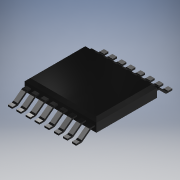
# Autodesk Inventor part: 16_pin_IC
Saved by Autodesk Inventor 2017 SP1 (Build 210196100, 196)
## iProperties
Created: 2016-08-29
Part Number: 16_pin_IC
Material: PBT Plastic
Document SubType Name: Modeling
Designer: jwrjc
Density: 1.31 g/cm^3
Appearance: Smooth - White
Author: jwrjc
Autodesk Inventor part; units mm, degrees
ref_plane "YZ Plane" through (0, 0, 0) normal (1, 0, 0) x (0, 1, 0)
ref_plane "XZ Plane" through (0, 0, 0) normal (0, 1, 0) x (-1, 0, 0)
ref_plane "XY Plane" through (0, 0, 0) normal (0, 0, 1) x (1, 0, 0)
sketch "Sketch1" plane through (0, 0, 0) normal (0, 0, 1) x (1, 0, 0)
  line L0 (-6.1646, -19.4392) -> (-11.1748, -19.4392)
  line L1 (-11.1748, -19.4392) -> (-11.1748, -23.673)
  line L2 (-11.1748, -23.673) -> (-6.1646, -23.673)
  line L3 (-6.1646, -23.673) -> (-6.1646, -19.4392)
  line L4 (-6.5748, -19.4392) -> (-6.2818, -19.4392)
  line L5 (-6.2818, -19.4392) -> (-6.2818, -18.2673)
  line L6 (-6.2818, -18.2673) -> (-6.5748, -18.2673)
  line L7 (-6.5748, -18.2673) -> (-6.5748, -19.4392)
  line L8 (-7.2047, -19.4392) -> (-6.8971, -19.4392)
  line L9 (-6.8971, -19.4392) -> (-6.8971, -18.2673)
  line L10 (-6.8971, -18.2673) -> (-7.2047, -18.2673)
  line L11 (-7.2047, -18.2673) -> (-7.2047, -19.4392)
  line L12 (-7.8347, -19.4392) -> (-7.5124, -19.4392)
  line L13 (-7.5124, -19.4392) -> (-7.5124, -18.2673)
  line L14 (-7.5124, -18.2673) -> (-7.8347, -18.2673)
  line L15 (-7.8347, -18.2673) -> (-7.8347, -19.4392)
  line L16 (-8.4939, -19.4392) -> (-8.1716, -19.4392)
  line L17 (-8.1716, -19.4392) -> (-8.1716, -18.2673)
  line L18 (-8.1716, -18.2673) -> (-8.4939, -18.2673)
  line L19 (-8.4939, -18.2673) -> (-8.4939, -19.4392)
  line L20 (-9.1824, -19.4392) -> (-8.8455, -19.4392)
  line L21 (-8.8455, -19.4392) -> (-8.8455, -18.2673)
  line L22 (-8.8455, -18.2673) -> (-9.1824, -18.2673)
  line L23 (-9.1824, -18.2673) -> (-9.1824, -19.4392)
  line L24 (-9.8124, -19.4392) -> (-9.4754, -19.4392)
  line L25 (-9.4754, -19.4392) -> (-9.4754, -18.2673)
  line L26 (-9.4754, -18.2673) -> (-9.8124, -18.2673)
  line L27 (-9.8124, -18.2673) -> (-9.8124, -19.4392)
  line L28 (-10.4569, -19.4392) -> (-10.1347, -19.4392)
  line L29 (-10.1347, -19.4392) -> (-10.1347, -18.2673)
  line L30 (-10.1347, -18.2673) -> (-10.4569, -18.2673)
  line L31 (-10.4569, -18.2673) -> (-10.4569, -19.4392)
  line L32 (-11.0429, -19.4392) -> (-10.7353, -19.4392)
  line L33 (-10.7353, -19.4392) -> (-10.7353, -18.2673)
  line L34 (-10.7353, -18.2673) -> (-11.0429, -18.2673)
  line L35 (-11.0429, -18.2673) -> (-11.0429, -19.4392)
  line L36 (-11.0429, -23.673) -> (-10.7353, -23.673)
  line L37 (-10.7353, -23.673) -> (-10.7353, -24.9622)
  line L38 (-10.7353, -24.9622) -> (-11.0429, -24.9622)
  line L39 (-11.0429, -24.9622) -> (-11.0429, -23.673)
  line L40 (-10.4569, -23.673) -> (-10.1347, -23.673)
  line L41 (-10.1347, -23.673) -> (-10.1347, -24.9622)
  line L42 (-10.1347, -24.9622) -> (-10.4569, -24.9622)
  line L43 (-10.4569, -24.9622) -> (-10.4569, -23.673)
  line L44 (-9.8124, -23.673) -> (-9.4754, -23.673)
  line L45 (-9.4754, -23.673) -> (-9.4754, -24.9622)
  line L46 (-9.4754, -24.9622) -> (-9.8124, -24.9622)
  line L47 (-9.8124, -24.9622) -> (-9.8124, -23.673)
  line L48 (-9.1824, -23.673) -> (-8.8455, -23.673)
  line L49 (-8.8455, -23.673) -> (-8.8455, -24.9622)
  line L50 (-8.8455, -24.9622) -> (-9.1824, -24.9622)
  line L51 (-9.1824, -24.9622) -> (-9.1824, -23.673)
  line L52 (-8.4939, -23.673) -> (-8.1716, -23.673)
  line L53 (-8.1716, -23.673) -> (-8.1716, -24.9622)
  line L54 (-8.1716, -24.9622) -> (-8.4939, -24.9622)
  line L55 (-8.4939, -24.9622) -> (-8.4939, -23.673)
  line L56 (-7.8347, -23.673) -> (-7.5124, -23.673)
  line L57 (-7.5124, -23.673) -> (-7.5124, -24.9622)
  line L58 (-7.5124, -24.9622) -> (-7.8347, -24.9622)
  line L59 (-7.8347, -24.9622) -> (-7.8347, -23.673)
  line L60 (-7.2047, -23.673) -> (-6.8971, -23.673)
  line L61 (-6.8971, -23.673) -> (-6.8971, -24.9622)
  line L62 (-6.8971, -24.9622) -> (-7.2047, -24.9622)
  line L63 (-7.2047, -24.9622) -> (-7.2047, -23.673)
  line L64 (-6.5748, -23.673) -> (-6.2818, -23.673)
  line L65 (-6.2818, -23.673) -> (-6.2818, -24.9622)
  line L66 (-6.2818, -24.9622) -> (-6.5748, -24.9622)
  line L67 (-6.5748, -24.9622) -> (-6.5748, -23.673)
  point P0 (0, 0)
  constraints: 132 end point, 33 parallel, 30 point on line, 16 horizontal, 16 perpendicular, 1 vertical, 22 other
extrude "Extrusion1" add sketch "Sketch1" along normal blind 1 contours L3 L2 L1 L0
extrude "Extrusion2" add sketch "Sketch1" along normal blind 0.6 contours L0 L7 L6 L5 | L65 L66 L67 L2 | L0 L11 L10 L9 | L61 L62 L63 L2 | L0 L15 L14 L13 | L57 L58 L59 L2 | L0 L19 L18 L17 | L53 L54 L55 L2 | L0 L23 L22 L21 | L49 L50 L51 L2 | L0 L27 L26 L25 | L45 L46 L47 L2 | L0 L31 L30 L29 | L41 L42 L43 L2 | L0 L35 L34 L33 | L37 L38 L39 L2
sketch "Sketch2" plane through (-11.0429, -19.4392, 0) normal (-1, 0, 0) x (0, 0, 1)
  line L0 (0, 0) -> (0, 1.172) projected
  line L1 (0.6, 1.172) -> (0.1113, 1.172)
  line L2 (0, 0) -> (0.599, 0)
  line L3 (0.6, 0.3044) -> (0.6, 1.172)
  line L4 (0.6, -4.2338) -> (0.6, -5.5229) projected
  line L5 (0, -4.2338) -> (0, -5.5229) projected
  line L6 (0.5, -4.2338) -> (0, -4.2338)
  line L7 (0, -4.2338) -> (0, -5.1366)
  line L8 (0.1113, -5.5229) -> (0.6, -5.5229)
  line L9 (0.6, -5.5229) -> (0.6, -4.5423)
  line L10 (0, 1.172) -> (0.6, 1.172) projected
  line L11 (0.1113, 1.172) -> (0.1113, 0.7931)
  line L12 (0.1113, 0.7931) -> (0.6, 0.3044)
  line L13 (0.6, 0) -> (0.6, 1.172) projected
  line L14 (0.6, 0) -> (0.5, 0)
  line L15 (0, 0) -> (1, 0) projected
  line L16 (0.5, 0) -> (0.5, 0.2353)
  line L17 (0.5, 0.2353) -> (0, 0.7353)
  line L18 (0, -5.5229) -> (0.6, -5.5229) projected
  line L19 (0.1113, -5.5229) -> (0.1113, -5.1962)
  line L20 (0.1113, -5.1962) -> (0.6, -4.5423)
  line L21 (0.6, -4.2338) -> (0.6, -4.2828)
  line L22 (0, -4.2338) -> (1, -4.2338) projected
  line L23 (0.5, -4.2338) -> (0.5, -4.4676)
  line L24 (0.5, -4.4676) -> (0, -5.1366)
  line L25 (0, 1.1726) -> (0, 1.172)
  line L26 (0, 0.7353) -> (0, 0)
  line L27 (0, 0.7353) -> (0.5, 0.2353)
  line L28 (0.5, 0.2353) -> (0.5, 0)
  line L29 (0.5, 0) -> (0, 0)
  line L30 (0, 0) -> (0, 0.7353)
  point P0 (0, 19.4392)
  constraints: 47 end point, 10 point on line, 7 parallel, 4 perpendicular, 3 collinear, 2 horizontal, 2 midpoint, 2 vertical
extrude "Extrusion3" cut sketch "Sketch2" against normal blind 4.9 contours L0 L17 L16 L2 | L1 L3 L12 L11 | L23 L24 L5 L6 | L4 L8 L19 L20
fillet "Fillet1" radius 0.2 64 edges at (-6.4283, -18.6461, 0.1113) (-7.0509, -18.6461, 0.1113) (-7.6735, -18.6461, 0.1113) (-8.3327, -18.6461, 0.1113) (-9.014, -18.6461, 0.1113) (-9.6439, -18.6461, 0.1113) (-10.2958, -18.6461, 0.1113) (-10.8891, -18.6461, 0.1113) (-10.8891, -19.1348, 0.6) (-10.2958, -19.1348, 0.6) (-9.6439, -19.1348, 0.6) (-9.014, -19.1348, 0.6) (-8.3327, -19.1348, 0.6) (-7.6735, -19.1348, 0.6) (-7.0509, -19.1348, 0.6) (-6.4283, -19.1348, 0.6) (-6.4283, -23.9816, 0.6) (-7.0509, -23.9816, 0.6) (-7.6735, -23.9816, 0.6) (-8.3327, -23.9816, 0.6) (-9.014, -23.9816, 0.6) (-9.6439, -23.9816, 0.6) (-10.2958, -23.9816, 0.6) (-10.8891, -23.9816, 0.6) (-10.8891, -23.9068, 0.5) (-10.2958, -23.9068, 0.5) (-9.6439, -23.9068, 0.5) (-9.014, -23.9068, 0.5) (-8.3327, -23.9068, 0.5) (-7.6735, -23.9068, 0.5) (-7.0509, -23.9068, 0.5) (-6.4283, -23.9068, 0.5) (-6.4283, -24.6354, 0.1113) (-6.4283, -24.5758, 0) (-7.0509, -24.6354, 0.1113) (-7.0509, -24.5758, 0) (-7.6735, -24.6354, 0.1113) (-7.6735, -24.5758, 0) (-8.3327, -24.6354, 0.1113) (-8.3327, -24.5758, 0) (-9.014, -24.6354, 0.1113) (-9.014, -24.5758, 0) (-9.6439, -24.6354, 0.1113) (-9.6439, -24.5758, 0) (-10.2958, -24.6354, 0.1113) (-10.2958, -24.5758, 0) (-10.8891, -24.6354, 0.1113) (-10.8891, -24.5758, 0) (-6.4283, -18.7039, 0) (-7.0509, -18.7039, 0) (-7.6735, -18.7039, 0) (-8.3327, -18.7039, 0) (-9.014, -18.7039, 0) (-9.6439, -18.7039, 0) (-10.2958, -18.7039, 0) (-10.8891, -18.7039, 0) (-10.8891, -19.2039, 0.5) (-10.2958, -19.2039, 0.5) (-9.6439, -19.2039, 0.5) (-9.014, -19.2039, 0.5) (-8.3327, -19.2039, 0.5) (-7.6735, -19.2039, 0.5) (-7.0509, -19.2039, 0.5) (-6.4283, -19.2039, 0.5)
chamfer "Chamfer1" distance 0.2 angle 45 8 edges at (-8.6697, -19.4392, 1) (-8.6697, -23.673, 1) (-6.1646, -21.5561, 1) (-11.1748, -21.5561, 1) (-8.6697, -19.4392, 0) (-11.1748, -21.5561, 0) (-6.1646, -21.5561, 0) (-8.6697, -23.673, 0)
body "Solid1"
